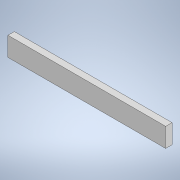
# Autodesk Inventor part: PrintHeadLoadPlate
Saved by Autodesk Inventor 2021 (Build 250183000, 183)
## iProperties
Created: 2021-10-26
Part Number: PrintHeadLoadPlate
Material: Generic
Document SubType Name: Sheet Metal
Designer: Unit-005
Density: 1 g/cm^3
Sheet Metal Rule: Default
Appearance: Default
Author: Unit-005
Autodesk Inventor part; units mm, degrees
ref_plane "YZ Plane" through (0, 0, 0) normal (1, 0, 0) x (0, 1, 0)
ref_plane "XZ Plane" through (0, 0, 0) normal (0, 1, 0) x (-1, 0, 0)
ref_plane "XY Plane" through (0, 0, 0) normal (0, 0, 1) x (1, 0, 0)
sketch "Sketch1" plane through (0, 0, 0) normal (0, 0, 1) x (1, 0, 0)
  line L0 (-39.1795, 4.7625) -> (39.1795, 4.7625)
  line L1 (39.1795, 4.7625) -> (39.1795, -4.7625)
  line L2 (39.1795, -4.7625) -> (-39.1795, -4.7625)
  line L3 (-39.1795, -4.7625) -> (-39.1795, 4.7625)
  line L4 (-39.1795, 4.7625) -> (39.1795, -4.7625) construction
  line L5 (39.1795, 4.7625) -> (-39.1795, -4.7625) construction
  point P0 (0, 0)
  dimension "d0" = 78.359
  dimension "d1" = 9.525
  constraints: 12 end point, 2 midpoint, 2 parallel, 1 horizontal, 1 perpendicular
  measures "d0" distance of L1.end L2.end
  measures "d1" distance of L0.end L1.end
extrude "Extrusion1" add sketch "Sketch1" along normal blind 3.175
sketch "Sketch2" plane through (0, 0, 0) normal (0, 0, -1) x (-1, 0, 0)
  line L0 (-54.8513, 0) -> (54.8513, 0) projected
  line L1 (0, -6.6675) -> (0, 6.6675) projected
  line L2 (39.1795, -4.7625) -> (-39.1795, -4.7625) projected
  line L3 (39.1795, 4.7625) -> (39.1795, -4.7625) projected
  line L4 (-39.1795, 4.7625) -> (39.1795, 4.7625) projected
  line L5 (-39.1795, -4.7625) -> (-39.1795, 4.7625) projected
  circle A0 centre (0, 2.6797) radius 1.5875
  point P0 (0, 0)
  dimension "d4" = 3.175
  dimension "d5" = 2.0828
  constraints: 1 centre point, 1 point on line
  measures "d4" diameter of A0
  measures "d5" distance from line of L4 A0.centre
extrude "Extrusion2" cut sketch "Sketch2" against normal blind 0.7937 contours A0 L1 | L1 A0
pattern_linear "Rectangular Pattern1" count 11 spacing 6.35 along (1, 0, 0) of "Extrusion2" first direction both ways yes
equation "\"BendRadius\" = Thickness"
equation "\"BendReliefWidth\" = Thickness"
equation "\"BendReliefDepth\" = 0.5 * Thickness"
equation "\"CornerReliefSize\" = 4 * Thickness"
equation "\"MinimumRemnant\" = 2 * Thickness"
equation "\"TransitionRadius\" = BendRadius"
equation "\"JacobiRadiusSize\" = BendRadius"
equation "\"GapSize\" = Thickness"
equation "\"Thickness\" = 3.048"
body "Solid1"
